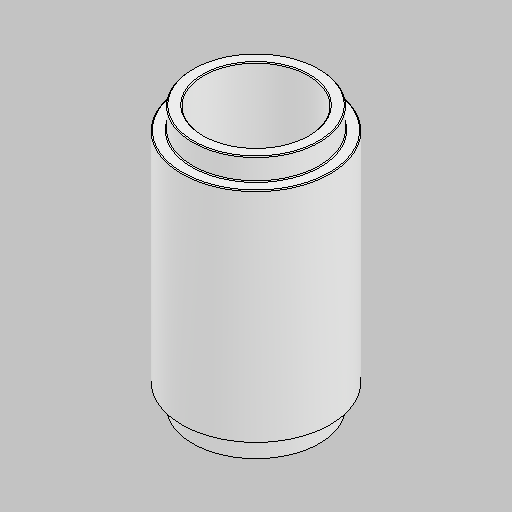
# Autodesk Inventor part: chamber_nipple03
Saved by Autodesk Inventor 2026 (Build 300175050, 175E)
## iProperties
Created: 2025-11-12
Part Number: chamber_nipple03
Material: ABS Plastic
Document SubType Name: Modeling
Designer: haru8
Density: 1.06 g/cm^3
Appearance: Smooth - White
Author: haru8
Autodesk Inventor part; units mm, degrees
ref_plane "YZ Plane" through (0, 0, 0) normal (1, 0, 0) x (0, 1, 0)
ref_plane "XZ Plane" through (0, 0, 0) normal (0, 1, 0) x (-1, 0, 0)
ref_plane "XY Plane" through (0, 0, 0) normal (0, 0, 1) x (1, 0, 0)
sketch "スケッチ1" plane through (0, 0, 0) normal (1, 0, 0) x (0, 1, 0)
  line L0 (-60, 29) -> (-50, 29)
  line L1 (-50, 29) -> (-50, 34)
  line L2 (-50, 34) -> (50, 34)
  line L3 (50, 34) -> (50, 29)
  line L4 (50, 29) -> (60, 29)
  line L5 (-60, 29) -> (-60, 24)
  line L6 (-60, 24) -> (60, 24)
  line L7 (-60, 0) -> (60, 0)
  line L8 (60, 29) -> (60, 24)
  point P0 (0, 0)
  point P1 (0, 0)
  dimension "d3" = 100
  dimension "d17" = 120
  dimension "d18" = 68
  dimension "d19" = 58
  dimension "d20" = 48
  constraints: 18 end point, 3 perpendicular, 3 vertical, 2 horizontal, 2 vertical alignment, 1 coincident, 1 collinear, 1 horizontal alignment, 1 midpoint
  measures "d3" distance of L1.end L2.end
  measures "d17" distance of L5.end L6.end
  measures "d18" diameter of L2 L7
  measures "d19" diameter of L4 L7
  measures "d20" diameter of L6 L7
revolve "回転1" add sketch "スケッチ1" angle 360 about axis through (0, -60, 0) along (0, 1, 0)
chamfer "Chamfer1" distance 0.4 angle 45 5 edges at (0, -60, -24) (0, 60, -24) (0, 60, -29) (0, 50, -29) (0, 50, -34)
